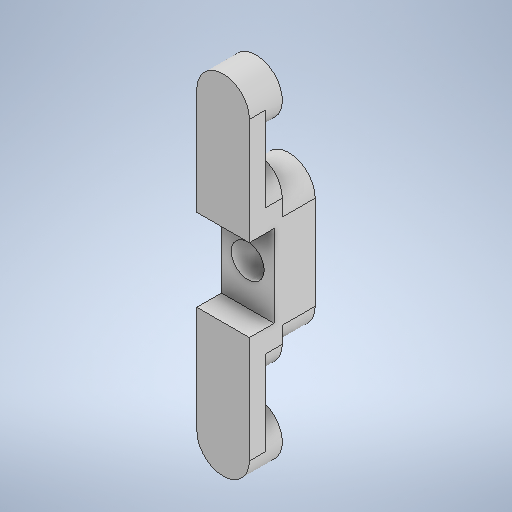
# Autodesk Inventor part: Button Cap
Saved by Autodesk Inventor 2026 (Build 300175050, 175E)
## iProperties
Created: 2025-07-10
Part Number: Button Cap
Material: Generic
Document SubType Name: Modeling
Designer: Jochen Alt
Density: 1 g/cm^3
Appearance: Default
Author: Jochen Alt
Autodesk Inventor part; units mm, degrees
ref_plane "YZ Plane" through (0, 0, 0) normal (1, 0, 0) x (0, 1, 0)
ref_plane "XZ Plane" through (0, 0, 0) normal (0, 1, 0) x (-1, 0, 0)
ref_plane "XY Plane" through (0, 0, 0) normal (0, 0, 1) x (1, 0, 0)
sketch "Sketch1" plane through (0, 0, 0) normal (0, 0, 1) x (1, 0, 0)
  line L0 (-2.31, 0) -> (2.31, 0) construction
  line L1 (0, 14.84) -> (0, -14.84) construction
  line L2 (0, 2.85) -> (0, -2.85) construction
  line L3 (-1.6, 2.85) -> (-1.6, -2.85)
  line L4 (1.6, -2.85) -> (1.6, 2.85)
  arc A0 (1.6, 2.85) -> (-1.6, 2.85) centre (0, 2.85) ccw
  arc A1 (-1.6, -2.85) -> (1.6, -2.85) centre (0, -2.85) ccw
  circle A2 centre (0, 0) radius 1
  line L5 (-1.6, 2.85) -> (-1.6, 9)
  arc A3 (1.6, 9) -> (-1.6, 9) centre (0, 9) ccw
  line L6 (1.6, 9) -> (1.6, 2.85)
  line L7 (-1.6, 2.85) -> (-1.6, 3.5)
  line L8 (1.6, 2.85) -> (1.6, 3.5)
  arc A4 (-1.6, 9) -> (1.6, 9) centre (0, 9) ccw
  line L9 (-1.6, -2.85) -> (-1.6, -9)
  arc A5 (-1.6, -9) -> (1.6, -9) centre (0, -9) ccw
  line L10 (1.6, -9) -> (1.6, -2.85)
  line L11 (-1.6, -2.85) -> (-1.6, -3.5)
  line L12 (1.6, -2.85) -> (1.6, -3.5)
  arc A6 (1.6, -9) -> (-1.6, -9) centre (0, -9) ccw
  line L13 (-1.6, 2.5) -> (1.6, 2.5)
  line L14 (-1.6, -2.5) -> (1.6, -2.5)
  arc A7 (-1.6, -3.85) -> (1.6, -3.85) centre (0, -3.85) ccw
  arc A8 (1.6, 3.85) -> (-1.6, 3.85) centre (0, 3.85) ccw
  point P0 (0, 4.45)
  point P1 (0, -4.45)
  point P2 (1.65, -3)
  point P3 (1.6008, -3)
  point P4 (-1.6008, -3)
  point P5 (-1.65, -3)
  point P6 (1.6, -2.85)
  point P7 (-1.6, -2.85)
  point P8 (-1.65, 3)
  point P9 (-1.6008, 3)
  point P10 (1.6008, 3)
  point P11 (1.65, 3)
  dimension "d2" = 2
  dimension "d16" = 2.5
  dimension "d17" = 8.9
  dimension "d18" = 3.2
  dimension "d22" = 1
  constraints: 28 end point, 20 point on circle, 11 point on line, 9 centre point, 8 symmetric about line, 8 tangent, 4 vertical, 2 coincident, 2 perpendicular, 1 midpoint, 1 parallel, 5 other
  measures "d2" diameter of A2
  measures "d16" distance from line of L13 point (0, 0)
  measures "d17" distance of point (0, 4.45) point (0, -4.45)
  measures "d18" distance between parallel lines of L3 L4
  measures "d22" distance of L2.end A7.centre
extrude "Extrusion1" add sketch "Sketch1" along normal blind 1 contours A0 L4 L13 L3 | L13 L4 L14 L3 | L14 L4 A1 L3 | A2
extrude "Extrusion2" add sketch "Sketch1" along normal blind 1.5 from surface at 1 contours A0 L4 L13 L3 | L13 L4 L14 L3 | L14 L4 A1 L3
extrude "Extrusion3" add sketch "Sketch1" along normal blind 0.5 from surface at 2.5 contours A0 L4 L13 L3 | L14 L4 A1 L3
extrude "Extrusion4" add sketch "Sketch1" along normal blind 1 from surface at 3 contours A0 L4 L13 L3 | L5 A8 L6 A0 | L14 L4 A1 L3 | L5 A4 L6 A8 | A1 L10 A7 L9 | A3 A4 | A7 L10 A6 L9 | A6 A5
extrude "Extrusion5" add sketch "Sketch1" against normal blind 1 from surface at 3 contours A3 A4 | A6 A5
extrude "Extrusion6" add sketch "Sketch1" against normal blind 1 from surface at 3 contours L5 A8 L6 A0 | A1 L10 A7 L9
body "Solid1"
